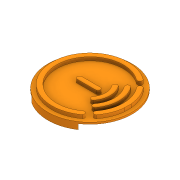
# Autodesk Inventor part: Scanner-Kapak
Saved by Autodesk Inventor 2020.3 (Build 243373000, 373)
## iProperties
Created: 2021-08-31
Part Number: Scanner-Kapak
Material: Generic
Document SubType Name: Modeling
Designer: Yusuf
Mass: 3.0014 g
Surface Area: 48.261 cm^2
Volume: 3.0014 cm^3
Density: 1 g/cm^3
Appearance: Orange
Author: Yusuf
Autodesk Inventor part; units mm, degrees
ref_plane "YZ Plane" through (0, 0, 0) normal (1, 0, 0) x (0, 1, 0)
ref_plane "XZ Plane" through (0, 0, 0) normal (0, 1, 0) x (-1, 0, 0)
ref_plane "XY Plane" through (0, 0, 0) normal (0, 0, 1) x (1, 0, 0)
sketch "Sketch1" plane through (0, 0, 0) normal (0, 1, 0) x (-1, 0, 0)
  circle A0 centre (0, 0) radius 24
  circle A1 centre (0, 0) radius 22
  dimension "d0" = 48
  dimension "d2" = 2
  constraints: 2 centre point, 2 coincident
  measures "d0" diameter of A0
  measures "d2" radial gap between concentric circles of A0 A1
extrude "Extrusion1" add sketch "Sketch1" along normal blind 4
sketch "Sketch2" plane through (0, 4, 0) normal (0, 1, 0) x (1, 0, 0)
  circle A0 centre (0, 0) radius 24
  circle A1 centre (0, 0) radius 22
  circle A2 centre (0, 0) radius 20
  circle A3 centre (0, 0) radius 17
  circle A4 centre (0, 0) radius 14
  circle A5 centre (0, 0) radius 11
  circle A6 centre (0, 0) radius 7
  circle A7 centre (0, 0) radius 4
  dimension "d10" = 40
  dimension "d11" = 48
  dimension "d12" = 44
  dimension "d13" = 34
  dimension "d14" = 28
  dimension "d15" = 22
  dimension "d16" = 14
  dimension "d17" = 8
  constraints: 8 centre point, 8 coincident
  measures "d10" diameter of A2
  measures "d11" diameter of A0
  measures "d12" diameter of A1
  measures "d13" diameter of A3
  measures "d14" diameter of A4
  measures "d15" diameter of A5
  measures "d16" diameter of A6
  measures "d17" diameter of A7
extrude "Extrusion2" add sketch "Sketch2" against normal blind 1 contours A0 | A1 | A2 | A3 | A4 | A5 | A6 | A7
sketch "Sketch3" plane through (0, 0, 0) normal (0, -1, 0) x (1, 0, 0)
  line L0 (-30, 20) -> (30, 20)
  line L1 (30, 20) -> (30, -20)
  line L2 (30, -20) -> (-30, -20)
  line L3 (-30, -20) -> (-30, 20)
  line L4 (-30, 20) -> (30, -20) construction
  line L5 (30, 20) -> (-30, -20) construction
  point P0 (0, 0)
  dimension "d7" = 60
  dimension "d8" = 40
  constraints: 12 end point, 2 midpoint, 2 parallel, 1 horizontal, 1 perpendicular
  measures "d7" distance of L1.end L2.end
  measures "d8" distance of L0.end L1.end
sketch "Sketch4" plane through (0, 4, 0) normal (0, 1, 0) x (1, 0, 0)
  circle A0 centre (-0.0001, 0.0001) radius 21.6961
  circle A1 centre (-0.0001, 0.0001) radius 19.037
  circle A2 centre (-0.0001, 0.0001) radius 16.6196
  circle A3 centre (-0.0001, 0.0001) radius 11.5431
  circle A4 centre (-0.0001, 0.0001) radius 8.884
  circle A5 centre (-0.0001, 0.0001) radius 13.9605
  line L0 (-0.0001, 21.6962) -> (-0.0001, -21.696) construction
  line L1 (-0.0001, 0.0001) -> (16.9795, -13.5061)
  line L2 (-0.0001, 0.0001) -> (13.057, -17.3272)
  arc A6 (14.8984, -11.8507) -> (16.9795, -13.5061) centre (16.142, -12.4231) ccw
  line L3 (15.9389, -12.6784) -> (16.1106, -12.4626) construction
  arc A7 (10.9255, -8.6905) -> (13.0065, -10.3459) centre (12.1691, -9.2629) ccw
  arc A8 (6.9526, -5.5303) -> (9.0336, -7.1857) centre (8.1962, -6.1027) ccw
  arc A9 (13.057, -17.3272) -> (11.4567, -15.2035) centre (11.9307, -16.5111) ccw
  arc A10 (16.9795, 13.5062) -> (14.8983, 11.8508) centre (16.144, 12.4206) ccw
  line L4 (-0.0001, 0.0001) -> (16.9795, 13.5062)
  arc A11 (13.0065, 10.346) -> (10.9254, 8.6906) centre (12.1712, 9.2602) ccw
  arc A12 (9.0335, 7.1858) -> (6.9525, 5.5304) centre (8.1983, 6.1) ccw
  arc A13 (11.4566, 15.2036) -> (13.057, 17.3274) centre (11.9308, 16.5111) ccw
  line L5 (-0.0001, 0.0001) -> (13.057, 17.3274)
  line L6 (15.9389, 12.6785) -> (16.1126, 12.4601) construction
  line L7 (19.0369, 0.0001) -> (16.6195, 0.0001)
  line L8 (13.9604, 0.0001) -> (11.543, 0.0001)
  line L9 (8.8839, 0.0001) -> (-21.6962, 0.0001)
  line L10 (21.62, -21.5289) -> (21.62, 21.5289)
  line L11 (-0.0001, 0.0001) -> (35.6066, 0.0001)
  line L12 (4.8627, -1.3296) -> (-6.2016, -1.3296)
  line L13 (4.8627, 1.3297) -> (-6.2016, 1.3297)
  line L14 (3.3126, -1.3296) -> (3.3126, 1.3297)
  arc A14 (4.8627, -1.3296) -> (4.8627, 1.3297) centre (4.6178, 0.0001) ccw
  arc A15 (-6.2016, 1.3297) -> (-6.2016, -1.3296) centre (-5.9623, 0.0001) ccw
  point P0 (0, 0)
  point P1 (21.6199, 0.0001)
  point P2 (-0.0001, 21.529)
  point P3 (3.3126, 0.0001)
  point P4 (28.4358, 37.7355)
  point P5 (32.4077, 43.0065)
  point P6 (22.4217, 17.835)
  point P7 (17.2565, 13.7264)
  point P8 (32.2826, 25.6787)
  point P9 (27.1174, 21.5701)
  point P10 (53.6613, 4.5036)
  point P11 (42.1434, 33.5224)
  point P12 (36.9782, 29.4138)
  point P13 (53.6613, -4.5036)
  point P14 (9.0336, 7.1858)
  point P15 (6.9523, 5.5309)
  point P16 (13.0065, 10.346)
  point P17 (10.9252, 8.6911)
  point P18 (11.457, 15.2035)
  point P19 (21.62, -1.8147)
  point P20 (21.62, 1.8149)
  point P21 (14.8981, 11.8513)
  dimension "d18" = 38.074
  dimension "d19" = 2.6591
  dimension "d20" = 2.6591
  dimension "d21" = 2.6591
  dimension "d22" = 2.4174
  dimension "d23" = 2.4174
  dimension "d24" = 1.369
  dimension "d25" = 2.6593
  dimension "d26" = 1.352
  dimension "d27" = 1.351
  constraints: 31 point on circle, 30 end point, 19 point on line, 15 centre point, 6 coincident, 6 horizontal, 3 perpendicular, 2 equal radius, 2 horizontal alignment, 2 midpoint, 1 vertical, 1 vertical alignment, 9 other
  measures "d18" diameter of A1
  measures "d20" radial gap between concentric circles of A4 A3
  measures "d21" radial gap between concentric circles of A5 A2
  measures "d22" radial gap between concentric circles of A2 A1
  measures "d23" radial gap between concentric circles of A3 A5
  measures "d24" radius of A6
  measures "d25" distance between parallel lines of L13 L12
  measures "d26" radius of A14
  measures "d27" radius of A15
extrude "Extrusion3" add sketch "Sketch4" along normal blind 2 contours L4 A10 | A0 L10 L11 A1 L4 | L5 A1 L9 A0 | A13 L5 | L9 A1 L2 A0 | L10 A0 L1 A1 L11 | A2 L11 A5 L4 | L4 A11 | L2 A9 | L1 A6 | A2 L1 A5 L11 | A7 L1 | A3 L11 A4 L4 | L4 A12 | A3 L1 A4 L11 | A8 L1 | L13 L14 L9 L4 | L4 L5 L13 | L5 L9 A15 L13 | A14 L12 L14 L9 | L9 L14 L13 A14 | L9 L14 L12 L1 | L1 L12 L2 | L2 L12 A15 L9
extrude "Extrusion4" cut sketch "Sketch3" against normal up to surface (3 mm away)
body "Solid1"
